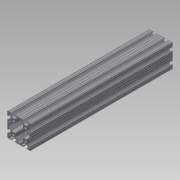
# Autodesk Inventor part: 2020
Saved by Autodesk Inventor 2013 (Build 170138000, 138)
## iProperties
Created: 2014-04-23
Part Number: 2020
Material: Generic
Document SubType Name: Modeling
Density: 1 g/cm^3
Vendor: 80/20 Inc.
Engineer: Ross Bowman
Designer: Ross Bowman
Catalog Web Link: 8020.net
Company: 80/20 Inc.
Author: Ross Bowman
Keywords: 80/20 , 8020 , T-Slot , Extrusion
Material: 6105-T5 Aluminum
Autodesk Inventor part; units mm, degrees
ref_plane "YZ Plane" through (0, 0, 0) normal (1, 0, 0) x (0, 1, 0)
ref_plane "XZ Plane" through (0, 0, 0) normal (0, 1, 0) x (-1, 0, 0)
ref_plane "XY Plane" through (0, 0, 0) normal (0, 0, 1) x (1, 0, 0)
sketch "Sketch1" plane through (0, 0, 0) normal (0, 0, 1) x (1, 0, 0)
  circle A0 centre (12.7, -12.7) radius 2.6035
  arc A1 (-1.9878, -21.7759) -> (0, -22.6304) centre (0.0777, -19.7104) ccw
  line L0 (-7.684, -16.0797) -> (-1.9878, -21.7759)
  arc A2 (-8.3312, -14.5171) -> (-7.684, -16.0797) centre (-6.1214, -14.5171) ccw
  line L1 (-8.3312, -10.3886) -> (-8.3312, -14.5171)
  arc A3 (-8.3312, -10.3886) -> (-10.541, -8.1788) centre (-10.541, -10.3886) ccw
  line L2 (-14.8165, -8.1788) -> (-10.541, -8.1788)
  arc A4 (-16.3772, -7.5334) -> (-14.8165, -8.1788) centre (-14.8165, -5.969) ccw
  line L3 (-21.7734, -2.1502) -> (-16.3772, -7.5334)
  arc A5 (-22.6314, -0.0822) -> (-21.7734, -2.1502) centre (-19.7104, -0.0822) ccw
  line L4 (-22.6314, 0.0822) -> (-22.6314, -0.0822)
  arc A6 (-21.7734, 2.1502) -> (-22.6314, 0.0822) centre (-19.7104, 0.0822) ccw
  line L5 (-16.3772, 7.5334) -> (-21.7734, 2.1502)
  arc A7 (-14.8165, 8.1788) -> (-16.3772, 7.5334) centre (-14.8165, 5.969) ccw
  line L6 (-10.541, 8.1788) -> (-14.8165, 8.1788)
  arc A8 (-10.541, 8.1788) -> (-8.3312, 10.3886) centre (-10.541, 10.3886) ccw
  line L7 (-8.3312, 14.5171) -> (-8.3312, 10.3886)
  arc A9 (-7.684, 16.0797) -> (-8.3312, 14.5171) centre (-6.1214, 14.5171) ccw
  line L8 (-1.7956, 21.9681) -> (-7.684, 16.0797)
  arc A10 (0, 22.8111) -> (-1.7956, 21.9681) centre (0.2699, 19.9026) ccw
  arc A11 (1.7956, 21.9681) -> (0, 22.8111) centre (-0.2699, 19.9026) ccw
  line L9 (7.684, 16.0797) -> (1.7956, 21.9681)
  arc A12 (8.3312, 14.5171) -> (7.684, 16.0797) centre (6.1214, 14.5171) ccw
  line L10 (8.3312, 10.389) -> (8.3312, 14.5171)
  arc A13 (8.3312, 10.389) -> (10.541, 8.1792) centre (10.541, 10.389) ccw
  line L11 (14.8161, 8.1792) -> (10.541, 8.1792)
  arc A14 (16.3768, 7.5339) -> (14.8161, 8.1792) centre (14.8161, 5.9694) ccw
  line L12 (21.7734, 2.1502) -> (16.3768, 7.5339)
  arc A15 (22.6314, 0.0822) -> (21.7734, 2.1502) centre (19.7104, 0.0822) ccw
  line L13 (22.6314, -0.0822) -> (22.6314, 0.0822)
  arc A16 (21.7734, -2.1502) -> (22.6314, -0.0822) centre (19.7104, -0.0822) ccw
  line L14 (16.3772, -7.5334) -> (21.7734, -2.1502)
  arc A17 (14.8165, -8.1788) -> (16.3772, -7.5334) centre (14.8165, -5.969) ccw
  line L15 (10.541, -8.1788) -> (14.8165, -8.1788)
  arc A18 (10.541, -8.1788) -> (8.3312, -10.3886) centre (10.541, -10.3886) ccw
  line L16 (8.3312, -14.5171) -> (8.3312, -10.3886)
  arc A19 (7.684, -16.0797) -> (8.3312, -14.5171) centre (6.1214, -14.5171) ccw
  line L17 (1.9878, -21.7759) -> (7.684, -16.0797)
  arc A20 (0, -22.6304) -> (1.9878, -21.7759) centre (-0.0777, -19.7104) ccw
  circle A21 centre (-12.7, -12.7) radius 2.6035
  circle A22 centre (-12.7, 12.7) radius 2.6035
  circle A23 centre (12.7, 12.7) radius 2.6035
  arc A24 (7.4579, -25.3998) -> (6.4535, -25.3998) centre (6.9557, -25.3232) ccw
  line L18 (7.4579, -25.3998) -> (8.4051, -25.3998)
  arc A25 (8.4051, -25.3998) -> (9.4615, -24.3585) centre (8.4201, -24.3585) ccw
  line L19 (9.4615, -24.3585) -> (9.4615, -24.2315)
  arc A26 (9.4615, -24.2315) -> (8.4051, -23.1902) centre (8.4201, -24.2315) ccw
  line L20 (8.4051, -23.1902) -> (6.0878, -23.1902)
  arc A27 (5.388, -21.5008) -> (6.0878, -23.1902) centre (6.0878, -22.2006) ccw
  line L21 (5.388, -21.5008) -> (8.763, -18.1257)
  arc A28 (11.0081, -17.1958) -> (8.763, -18.1257) centre (11.0081, -20.3708) ccw
  line L22 (11.0081, -17.1958) -> (14.3919, -17.1958)
  arc A29 (16.637, -18.1257) -> (14.3919, -17.1958) centre (14.3919, -20.3708) ccw
  line L23 (16.637, -18.1257) -> (20.012, -21.5008)
  arc A30 (19.2977, -23.1901) -> (20.012, -21.5008) centre (19.3122, -22.2006) ccw
  line L24 (19.2977, -23.1901) -> (16.9799, -23.1901)
  arc A31 (16.9799, -23.1901) -> (15.9385, -24.2315) centre (16.9799, -24.2315) ccw
  line L25 (15.9385, -24.2315) -> (15.9385, -24.3585)
  arc A32 (15.9385, -24.3585) -> (16.9949, -25.3998) centre (16.9799, -24.3585) ccw
  line L26 (16.9949, -25.3998) -> (18.134, -25.3998)
  arc A33 (19.1384, -25.3998) -> (18.134, -25.3998) centre (18.6362, -25.3232) ccw
  line L27 (19.1384, -25.3998) -> (22.4132, -25.3998)
  arc A34 (23.4176, -25.3998) -> (22.4132, -25.3998) centre (22.9154, -25.3232) ccw
  line L28 (23.4176, -25.3998) -> (23.4501, -25.3998)
  arc A35 (23.4501, -25.3998) -> (25.4, -23.2975) centre (23.2918, -23.2975) ccw
  line L29 (25.4, -23.2975) -> (25.4, -23.2686)
  arc A36 (25.4, -22.2526) -> (25.4, -23.2686) centre (25.4, -22.7606) ccw
  line L30 (25.4, -22.2526) -> (25.4, -19.0252)
  arc A37 (25.4, -18.0092) -> (25.4, -19.0252) centre (25.4, -18.5172) ccw
  line L31 (25.4, -18.0092) -> (25.4, -16.916)
  arc A38 (25.4, -16.916) -> (24.3586, -15.8746) centre (24.3586, -16.916) ccw
  line L32 (24.3586, -15.8746) -> (24.2316, -15.8746)
  arc A39 (24.2316, -15.8746) -> (23.1902, -16.916) centre (24.2316, -16.916) ccw
  line L33 (23.1902, -16.916) -> (23.1902, -19.101)
  arc A40 (21.4558, -19.8194) -> (23.1902, -19.101) centre (22.1742, -19.101) ccw
  line L34 (21.4558, -19.8194) -> (18.2781, -16.6418)
  arc A41 (17.3482, -14.3967) -> (18.2781, -16.6418) centre (20.5232, -14.3967) ccw
  line L35 (17.3482, -14.3967) -> (17.3482, -11.0035)
  arc A42 (18.2808, -8.7557) -> (17.3482, -11.0035) centre (20.5232, -11.0035) ccw
  line L36 (18.2808, -8.7557) -> (21.4566, -5.5875)
  arc A43 (23.1902, -6.3068) -> (21.4566, -5.5875) centre (22.1742, -6.3068) ccw
  line L37 (23.1902, -6.3068) -> (23.1902, -8.484)
  arc A44 (23.1902, -8.484) -> (24.2316, -9.5254) centre (24.2316, -8.484) ccw
  line L38 (24.2316, -9.5254) -> (24.3586, -9.5254)
  arc A45 (24.3586, -9.5254) -> (25.4, -8.484) centre (24.3586, -8.484) ccw
  line L39 (25.4, -8.484) -> (25.4, -7.3277)
  arc A46 (25.4, -6.3117) -> (25.4, -7.3277) centre (25.4, -6.8197) ccw
  line L40 (25.4, -6.3117) -> (25.4, -3.0843)
  arc A47 (25.4, -2.0683) -> (25.4, -3.0843) centre (25.4, -2.5763) ccw
  line L41 (25.4, -2.0683) -> (25.4, 2.0683)
  arc A48 (25.4, 3.0843) -> (25.4, 2.0683) centre (25.4, 2.5763) ccw
  line L42 (25.4, 3.0843) -> (25.4, 6.3117)
  arc A49 (25.4, 7.3277) -> (25.4, 6.3117) centre (25.4, 6.8197) ccw
  line L43 (25.4, 7.3277) -> (25.4, 8.484)
  arc A50 (25.4, 8.484) -> (24.3586, 9.5254) centre (24.3586, 8.484) ccw
  line L44 (24.3586, 9.5254) -> (24.2316, 9.5254)
  arc A51 (24.2316, 9.5254) -> (23.1902, 8.484) centre (24.2316, 8.484) ccw
  line L45 (23.1902, 8.484) -> (23.1902, 6.3068)
  arc A52 (21.4566, 5.5875) -> (23.1902, 6.3068) centre (22.1742, 6.3068) ccw
  line L46 (21.4566, 5.5875) -> (18.2808, 8.7557)
  arc A53 (17.3482, 11.0035) -> (18.2808, 8.7557) centre (20.5232, 11.0035) ccw
  line L47 (17.3482, 11.0035) -> (17.3482, 14.3967)
  arc A54 (18.2781, 16.6418) -> (17.3482, 14.3967) centre (20.5232, 14.3967) ccw
  line L48 (18.2781, 16.6418) -> (21.4558, 19.8194)
  arc A55 (23.1902, 19.101) -> (21.4558, 19.8194) centre (22.1742, 19.101) ccw
  line L49 (23.1902, 19.101) -> (23.1902, 16.916)
  arc A56 (23.1902, 16.916) -> (24.2316, 15.8746) centre (24.2316, 16.916) ccw
  line L50 (24.2316, 15.8746) -> (24.3586, 15.8746)
  arc A57 (24.3586, 15.8746) -> (25.4, 16.916) centre (24.3586, 16.916) ccw
  line L51 (25.4, 16.916) -> (25.4, 18.0092)
  arc A58 (25.4, 19.0252) -> (25.4, 18.0092) centre (25.4, 18.5172) ccw
  line L52 (25.4, 19.0252) -> (25.4, 22.2526)
  arc A59 (25.4, 23.2686) -> (25.4, 22.2526) centre (25.4, 22.7606) ccw
  line L53 (25.4, 23.2686) -> (25.4, 23.2975)
  arc A60 (25.4, 23.2975) -> (23.4501, 25.3998) centre (23.2918, 23.2975) ccw
  line L54 (23.4501, 25.3998) -> (23.4176, 25.3998)
  arc A61 (22.4132, 25.3998) -> (23.4176, 25.3998) centre (22.9154, 25.3232) ccw
  line L55 (22.4132, 25.3998) -> (19.1384, 25.3998)
  arc A62 (18.134, 25.3998) -> (19.1384, 25.3998) centre (18.6362, 25.3232) ccw
  line L56 (18.134, 25.3998) -> (16.9949, 25.3998)
  arc A63 (16.9949, 25.3998) -> (15.9385, 24.3585) centre (16.9799, 24.3585) ccw
  line L57 (15.9385, 24.3585) -> (15.9385, 24.2315)
  arc A64 (15.9385, 24.2315) -> (16.9799, 23.1901) centre (16.9799, 24.2315) ccw
  line L58 (16.9799, 23.1901) -> (19.2977, 23.1901)
  arc A65 (20.012, 21.5008) -> (19.2977, 23.1901) centre (19.3122, 22.2006) ccw
  line L59 (20.012, 21.5008) -> (16.637, 18.1257)
  arc A66 (14.3919, 17.1958) -> (16.637, 18.1257) centre (14.3919, 20.3708) ccw
  line L60 (14.3919, 17.1958) -> (11.0081, 17.1958)
  arc A67 (8.763, 18.1257) -> (11.0081, 17.1958) centre (11.0081, 20.3708) ccw
  line L61 (8.763, 18.1257) -> (5.388, 21.5008)
  arc A68 (6.0878, 23.1902) -> (5.388, 21.5008) centre (6.0878, 22.2006) ccw
  line L62 (6.0878, 23.1902) -> (8.4051, 23.1902)
  arc A69 (8.4051, 23.1902) -> (9.4615, 24.2315) centre (8.4201, 24.2315) ccw
  line L63 (9.4615, 24.2315) -> (9.4615, 24.3585)
  arc A70 (9.4615, 24.3585) -> (8.4051, 25.3998) centre (8.4201, 24.3585) ccw
  line L64 (8.4051, 25.3998) -> (7.4579, 25.3998)
  arc A71 (6.4535, 25.3998) -> (7.4579, 25.3998) centre (6.9557, 25.3232) ccw
  line L65 (6.4535, 25.3998) -> (3.2145, 25.3998)
  arc A72 (2.2101, 25.3998) -> (3.2145, 25.3998) centre (2.7123, 25.3232) ccw
  line L66 (2.2101, 25.3998) -> (-2.2101, 25.3998)
  arc A73 (-3.2145, 25.3998) -> (-2.2101, 25.3998) centre (-2.7123, 25.3232) ccw
  line L67 (-3.2145, 25.3998) -> (-6.4535, 25.3998)
  arc A74 (-7.4579, 25.3998) -> (-6.4535, 25.3998) centre (-6.9557, 25.3232) ccw
  line L68 (-7.4579, 25.3998) -> (-8.4051, 25.3998)
  arc A75 (-8.4051, 25.3998) -> (-9.4615, 24.3585) centre (-8.4201, 24.3585) ccw
  line L69 (-9.4615, 24.3585) -> (-9.4615, 24.2315)
  arc A76 (-9.4615, 24.2315) -> (-8.4051, 23.1902) centre (-8.4201, 24.2315) ccw
  line L70 (-8.4051, 23.1902) -> (-6.0878, 23.1902)
  arc A77 (-5.388, 21.5008) -> (-6.0878, 23.1902) centre (-6.0878, 22.2006) ccw
  line L71 (-5.388, 21.5008) -> (-8.763, 18.1257)
  arc A78 (-11.0081, 17.1958) -> (-8.763, 18.1257) centre (-11.0081, 20.3708) ccw
  line L72 (-11.0081, 17.1958) -> (-14.3919, 17.1958)
  arc A79 (-16.637, 18.1257) -> (-14.3919, 17.1958) centre (-14.3919, 20.3708) ccw
  line L73 (-16.637, 18.1257) -> (-20.012, 21.5008)
  arc A80 (-19.2977, 23.1901) -> (-20.012, 21.5008) centre (-19.3122, 22.2006) ccw
  line L74 (-19.2977, 23.1901) -> (-16.9799, 23.1901)
  arc A81 (-16.9799, 23.1901) -> (-15.9385, 24.2315) centre (-16.9799, 24.2315) ccw
  line L75 (-15.9385, 24.2315) -> (-15.9385, 24.3585)
  arc A82 (-15.9385, 24.3585) -> (-16.9949, 25.3998) centre (-16.9799, 24.3585) ccw
  line L76 (-16.9949, 25.3998) -> (-18.134, 25.3998)
  arc A83 (-19.1384, 25.3998) -> (-18.134, 25.3998) centre (-18.6362, 25.3232) ccw
  line L77 (-19.1384, 25.3998) -> (-22.4132, 25.3998)
  arc A84 (-23.4176, 25.3998) -> (-22.4132, 25.3998) centre (-22.9154, 25.3232) ccw
  line L78 (-23.4176, 25.3998) -> (-23.4501, 25.3998)
  arc A85 (-23.4501, 25.3998) -> (-25.4, 23.2975) centre (-23.2918, 23.2975) ccw
  line L79 (-25.4, 23.2975) -> (-25.4, 23.2686)
  arc A86 (-25.4, 22.2526) -> (-25.4, 23.2686) centre (-25.4, 22.7606) ccw
  line L80 (-25.4, 22.2526) -> (-25.4, 19.0252)
  arc A87 (-25.4, 18.0092) -> (-25.4, 19.0252) centre (-25.4, 18.5172) ccw
  line L81 (-25.4, 18.0092) -> (-25.4, 16.916)
  arc A88 (-25.4, 16.916) -> (-24.3586, 15.8746) centre (-24.3586, 16.916) ccw
  line L82 (-24.3586, 15.8746) -> (-24.2316, 15.8746)
  arc A89 (-24.2316, 15.8746) -> (-23.1902, 16.916) centre (-24.2316, 16.916) ccw
  line L83 (-23.1902, 16.916) -> (-23.1902, 19.101)
  arc A90 (-21.4558, 19.8194) -> (-23.1902, 19.101) centre (-22.1742, 19.101) ccw
  line L84 (-21.4558, 19.8194) -> (-18.2781, 16.6418)
  arc A91 (-17.3482, 14.3967) -> (-18.2781, 16.6418) centre (-20.5232, 14.3967) ccw
  line L85 (-17.3482, 14.3967) -> (-17.3482, 11.0035)
  arc A92 (-18.2808, 8.7557) -> (-17.3482, 11.0035) centre (-20.5232, 11.0035) ccw
  line L86 (-18.2808, 8.7557) -> (-21.4566, 5.5875)
  arc A93 (-23.1902, 6.3068) -> (-21.4566, 5.5875) centre (-22.1742, 6.3068) ccw
  line L87 (-23.1902, 6.3068) -> (-23.1902, 8.484)
  arc A94 (-23.1902, 8.484) -> (-24.2316, 9.5254) centre (-24.2316, 8.484) ccw
  line L88 (-24.2316, 9.5254) -> (-24.3586, 9.5254)
  arc A95 (-24.3586, 9.5254) -> (-25.4, 8.484) centre (-24.3586, 8.484) ccw
  line L89 (-25.4, 8.484) -> (-25.4, 7.3277)
  arc A96 (-25.4, 6.3117) -> (-25.4, 7.3277) centre (-25.4, 6.8197) ccw
  line L90 (-25.4, 6.3117) -> (-25.4, 3.0843)
  arc A97 (-25.4, 2.0683) -> (-25.4, 3.0843) centre (-25.4, 2.5763) ccw
  line L91 (-25.4, 2.0683) -> (-25.4, -2.0683)
  arc A98 (-25.4, -3.0843) -> (-25.4, -2.0683) centre (-25.4, -2.5763) ccw
  line L92 (-25.4, -3.0843) -> (-25.4, -6.3117)
  arc A99 (-25.4, -7.3277) -> (-25.4, -6.3117) centre (-25.4, -6.8197) ccw
  line L93 (-25.4, -7.3277) -> (-25.4, -8.484)
  arc A100 (-25.4, -8.484) -> (-24.3586, -9.5254) centre (-24.3586, -8.484) ccw
  line L94 (-24.3586, -9.5254) -> (-24.2316, -9.5254)
  arc A101 (-24.2316, -9.5254) -> (-23.1902, -8.484) centre (-24.2316, -8.484) ccw
  line L95 (-23.1902, -8.484) -> (-23.1902, -6.3068)
  arc A102 (-21.4566, -5.5875) -> (-23.1902, -6.3068) centre (-22.1742, -6.3068) ccw
  line L96 (-21.4566, -5.5875) -> (-18.2808, -8.7557)
  arc A103 (-17.3482, -11.0035) -> (-18.2808, -8.7557) centre (-20.5232, -11.0035) ccw
  line L97 (-17.3482, -11.0035) -> (-17.3482, -14.3967)
  arc A104 (-18.2781, -16.6418) -> (-17.3482, -14.3967) centre (-20.5232, -14.3967) ccw
  line L98 (-18.2781, -16.6418) -> (-21.4558, -19.8194)
  arc A105 (-23.1902, -19.101) -> (-21.4558, -19.8194) centre (-22.1742, -19.101) ccw
  line L99 (-23.1902, -19.101) -> (-23.1902, -16.916)
  arc A106 (-23.1902, -16.916) -> (-24.2316, -15.8746) centre (-24.2316, -16.916) ccw
  line L100 (-24.2316, -15.8746) -> (-24.3586, -15.8746)
  arc A107 (-24.3586, -15.8746) -> (-25.4, -16.916) centre (-24.3586, -16.916) ccw
  line L101 (-25.4, -16.916) -> (-25.4, -18.0092)
  arc A108 (-25.4, -19.0252) -> (-25.4, -18.0092) centre (-25.4, -18.5172) ccw
  line L102 (-25.4, -19.0252) -> (-25.4, -22.2526)
  arc A109 (-25.4, -23.2686) -> (-25.4, -22.2526) centre (-25.4, -22.7606) ccw
  line L103 (-25.4, -23.2686) -> (-25.4, -23.2975)
  arc A110 (-25.4, -23.2975) -> (-23.4501, -25.3998) centre (-23.2918, -23.2975) ccw
  line L104 (-23.4501, -25.3998) -> (-23.4176, -25.3998)
  arc A111 (-22.4132, -25.3998) -> (-23.4176, -25.3998) centre (-22.9154, -25.3232) ccw
  line L105 (-22.4132, -25.3998) -> (-19.1384, -25.3998)
  arc A112 (-18.134, -25.3998) -> (-19.1384, -25.3998) centre (-18.6362, -25.3232) ccw
  line L106 (-18.134, -25.3998) -> (-16.9949, -25.3998)
  arc A113 (-16.9949, -25.3998) -> (-15.9385, -24.3585) centre (-16.9799, -24.3585) ccw
  line L107 (-15.9385, -24.3585) -> (-15.9385, -24.2315)
  arc A114 (-15.9385, -24.2315) -> (-16.9799, -23.1901) centre (-16.9799, -24.2315) ccw
  line L108 (-16.9799, -23.1901) -> (-19.2977, -23.1901)
  arc A115 (-20.012, -21.5008) -> (-19.2977, -23.1901) centre (-19.3122, -22.2006) ccw
  line L109 (-20.012, -21.5008) -> (-16.637, -18.1257)
  arc A116 (-14.3919, -17.1958) -> (-16.637, -18.1257) centre (-14.3919, -20.3708) ccw
  line L110 (-14.3919, -17.1958) -> (-11.0081, -17.1958)
  arc A117 (-8.763, -18.1257) -> (-11.0081, -17.1958) centre (-11.0081, -20.3708) ccw
  line L111 (-8.763, -18.1257) -> (-5.388, -21.5008)
  arc A118 (-6.0878, -23.1902) -> (-5.388, -21.5008) centre (-6.0878, -22.2006) ccw
  line L112 (-6.0878, -23.1902) -> (-8.4051, -23.1902)
  arc A119 (-8.4051, -23.1902) -> (-9.4615, -24.2315) centre (-8.4201, -24.2315) ccw
  line L113 (-9.4615, -24.2315) -> (-9.4615, -24.3585)
  arc A120 (-9.4615, -24.3585) -> (-8.4051, -25.3998) centre (-8.4201, -24.3585) ccw
  line L114 (-8.4051, -25.3998) -> (-7.4579, -25.3998)
  arc A121 (-6.4535, -25.3998) -> (-7.4579, -25.3998) centre (-6.9557, -25.3232) ccw
  line L115 (-6.4535, -25.3998) -> (-3.2145, -25.3998)
  arc A122 (-2.2101, -25.3998) -> (-3.2145, -25.3998) centre (-2.7123, -25.3232) ccw
  line L116 (-2.2101, -25.3998) -> (2.2101, -25.3998)
  arc A123 (3.2145, -25.3998) -> (2.2101, -25.3998) centre (2.7123, -25.3232) ccw
  line L117 (3.2145, -25.3998) -> (6.4535, -25.3998)
  point P0 (0, 0)
  constraints: 240 point on circle, 236 end point, 124 centre point
extrude "Extrusion1" add sketch "Sketch1" against normal blind 304.8
body "Solid1"
